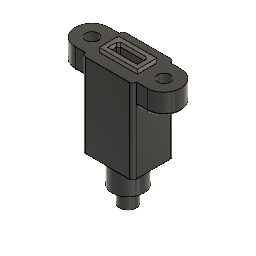
3258 microUSB panel mount (Autodesk Fusion 360 design; units mm, degrees)
Autodesk Fusion 360 part; units mm, degrees
sketch "Sketch1" plane through (0, 0, 0) normal (0, 0, 1) x (1, 0, 0)
  line L0 (4.5, -2.3) -> (-4.5, -2.3)
  line L1 (-4.5, -2.3) -> (-4.5, 2.3)
  line L2 (-4.5, 2.3) -> (4.5, 2.3)
  line L3 (4.5, 2.3) -> (4.5, -2.3)
  line L4 (4.5, -2.3) -> (-4.5, 2.3) construction
  line L5 (-4.5, -2.3) -> (4.5, 2.3) construction
  line L6 (3.5, -1.3) -> (-3.5, -1.3)
  line L7 (-3.5, -1.3) -> (-3.5, 1.3)
  line L8 (-3.5, 1.3) -> (3.5, 1.3)
  line L9 (3.5, 1.3) -> (3.5, -1.3)
  line L10 (6, -4.9) -> (-6, -4.9)
  line L11 (-6, -4.9) -> (-6, 4.9)
  line L12 (-6, 4.9) -> (6, 4.9)
  line L13 (6, 4.9) -> (6, -4.9)
  line L14 (6, -4.9) -> (-6, 4.9) construction
  line L15 (-6, -4.9) -> (6, 4.9) construction
  circle A0 centre (-8.5, 0) radius 1.5
  line L16 (-8.5, -4) -> (0, -4)
  arc A1 (0, -4) -> (0, 4) centre (0, 0) ccw
  line L17 (0, 4) -> (-8.5, 4)
  arc A2 (-8.5, 4) -> (-8.5, -4) centre (-8.5, 0) ccw
  line L18 (-8.5, 0) -> (0, 0) construction
  dimension "d1" = 9
  dimension "d2" = 4.6
  dimension "d3" = 1
  dimension "d4" = 12
  dimension "d5" = 9.8
  dimension "d6" = 3
  dimension "d7" = 8.5
  dimension "d8" = 8
  measures "d3" distance of L0
  measures "d6" diameter of A0
  measures "d7" distance of A1.centre
  measures "d8" diameter of A1
extrude "Extrude1" add sketch "Sketch1" against normal blind 19.8 contours L0 L2 L3 L10 L11 L12 L13 L16 A1 L17 | L0 L2 L3 A1 | L0 L1 L2 L11 L16 A1 L17 | L0 L1 L2 A1 | L6 L7 L8 L9 makes body 1
extrude "Extrude2" add sketch "Sketch1" along normal blind 1 separate body contours L0 L2 L3 A1 | L0 L1 L2 A1 makes body 2
fillet "Fillet1" radius 0.8 4 edges at (6, -4.9, -9.9) (-6, -4.9, -9.9) (-6, 4.9, -9.9) (6, 4.9, -9.9) on bodies 1
extrude "Extrude3" add sketch "Sketch1" against normal blind 5 contours L11 L16 L17 A2 bodies 1
mirror "Mirror1" about plane through (0, 0, 0) normal (1, 0, 0) of "Extrude3"
chamfer "Chamfer2" distance 0.5 angle 45 2 edges at (3.5, 1.3, 0.5) (-3.5, 1.3, 0.5) on bodies 2
fillet "Fillet2" radius 0.6 6 edges at (7.25, -4, -5) (12.5, 0, -5) (7.25, 4, -5) (-7.25, -4, -5) (-12.5, 0, -5) (-7.25, 4, -5) on bodies 1
sketch "Sketch2" plane through (0, 0, -19.8) normal (0, 0, -1) x (1, 0, 0)
  arc A0 (5.2, -4.9) -> (6, -4.1) centre (5.2, -4.1) ccw
  line L0 (6, -4.1) -> (6, 4.1)
  arc A1 (6, 4.1) -> (5.2, 4.9) centre (5.2, 4.1) ccw
  line L1 (5.2, 4.9) -> (-5.2, 4.9)
  arc A2 (-5.2, 4.9) -> (-6, 4.1) centre (-5.2, 4.1) ccw
  line L2 (-6, 4.1) -> (-6, -4.1)
  arc A3 (-6, -4.1) -> (-5.2, -4.9) centre (-5.2, -4.1) ccw
  line L3 (-5.2, -4.9) -> (5.2, -4.9)
  circle A4 centre (0, 0) radius 3.8
  circle A5 centre (0, 0) radius 2
  dimension "d20" = 7.6
  dimension "d21" = 4
  measures "d20" diameter of A4
  measures "d21" diameter of A5
extrude "Extrude4" add sketch "Sketch2" along normal blind 6 contours A4 | A5 bodies 1
extrude "Extrude5" add sketch "Sketch2" along normal blind 4 from surface at 6 contours A5 bodies 1
sketch "Sketch3" plane through (0, 0, 0) normal (0, 0, 1) x (-1, 0, 0)
  circle A0 centre (-8.5, 0) radius 1.5
  circle A1 centre (8.5, 0) radius 1.5
  arc A2 (-6, -4.1) -> (-5.2, -4.9) centre (-5.2, -4.1) ccw
  line L0 (-5.2, -4.9) -> (5.2, -4.9)
  arc A3 (5.2, -4.9) -> (6, -4.1) centre (5.2, -4.1) ccw
  line L1 (6, -4.1) -> (6, -4)
  line L2 (6, -4) -> (8.5, -4)
  arc A4 (8.5, -4) -> (8.5, 4) centre (8.5, 0) ccw
  line L3 (8.5, 4) -> (6, 4)
  line L4 (6, 4) -> (6, 4.1)
  arc A5 (6, 4.1) -> (5.2, 4.9) centre (5.2, 4.1) ccw
  line L5 (5.2, 4.9) -> (-5.2, 4.9)
  arc A6 (-5.2, 4.9) -> (-6, 4.1) centre (-5.2, 4.1) ccw
  line L6 (-6, 4.1) -> (-6, 4)
  line L7 (-6, 4) -> (-8.5, 4)
  arc A7 (-8.5, 4) -> (-8.5, -4) centre (-8.5, 0) ccw
  line L8 (-8.5, -4) -> (-6, -4)
  line L9 (-6, -4) -> (-6, -4.1)
  line L10 (3, -1.3) -> (-3, -1.3)
  line L11 (-3, -1.3) -> (-3.5, -0.8)
  line L12 (-3.5, -0.8) -> (-3.5, 1.3)
  line L13 (-3.5, 1.3) -> (3.5, 1.3)
  line L14 (3.5, 1.3) -> (3.5, -0.8)
  line L15 (3.5, -0.8) -> (3, -1.3)
  line L16 (-4.5, -2.3) -> (4.5, -2.3)
  line L17 (4.5, -2.3) -> (4.5, 2.3)
  line L18 (4.5, 2.3) -> (-4.5, 2.3)
  line L19 (-4.5, 2.3) -> (-4.5, -2.3)
extrude "Extrude6" cut sketch "Sketch3" against normal blind 2 contours L10 L11 L12 L13 L14 L15 bodies 1
equation "d7 = ( 17 / 2 ) * 1 mm"
